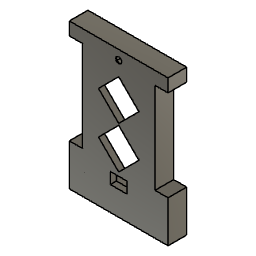
CAO Sablier face avant  v3 -42mm v1 (Autodesk Fusion 360 design; units mm, degrees)
Autodesk Fusion 360 part; units mm, degrees
sketch "Esquisse1" plane through (0, 0, 0) normal (0, 1, 0) x (1, 0, 0)
  line L0 (0, 0) -> (114, 0)
  line L1 (114, 0) -> (114, -150)
  line L2 (114, -150) -> (0, -150)
  line L3 (0, -150) -> (0, 0)
  line L4 (66.6, -23) -> (47.4, -23)
  line L5 (47.4, -23) -> (47.4, -10)
  line L6 (47.4, -10) -> (66.6, -10)
  line L7 (66.6, -10) -> (66.6, -23)
  line L8 (57, -122.669) -> (80.3345, -99.3345)
  line L9 (80.3345, -99.3345) -> (57, -76)
  line L10 (57, -76) -> (33.6655, -99.3345)
  line L11 (33.6655, -99.3345) -> (57, -122.669)
  line L12 (114, -75) -> (0, -75)
  line L13 (33.6655, -50.6655) -> (57, -27.331)
  line L14 (57, -27.331) -> (80.3345, -50.6655)
  line L15 (80.3345, -50.6655) -> (57, -74)
  line L16 (57, -74) -> (33.6655, -50.6655)
  line L17 (114, -135) -> (99, -135)
  line L18 (99, -135) -> (99, -30)
  line L19 (99, -30) -> (114, -30)
  line L20 (114, -30) -> (114, -135)
  line L21 (57, -150) -> (57, 0)
  line L22 (0, -135) -> (15, -135)
  line L23 (15, -135) -> (15, -30)
  line L24 (15, -30) -> (0, -30)
  point P0 (57, -23)
  point P1 (57, -150)
  point P2 (57, -75)
  dimension "d1" = 114
  dimension "d2" = 150
  dimension "d44" = 13
  dimension "d45" = 19.2
  dimension "d46" = 10
  dimension "d48" = 1
  dimension "d49" = 33
  dimension "d159" = 15
  dimension "d160" = 15
  dimension "d161" = 30
  constraint horizontal L0
  constraint vertical L1
  constraint horizontal L2
  constraint vertical L3
  constraint coincident L0.start L3.end
  constraint horizontal L4
  constraint vertical L5
  constraint horizontal L6
  constraint vertical L7
  constraint midpoint L4 P0
  constraint midpoint L2 P1
  constraint vertical P0 P1
  constraint perpendicular L8 L9
  constraint parallel L8 L10
  constraint parallel L9 L11
  constraint vertical L8.start L9.end
  constraint horizontal L8.end L10.end
  constraint vertical P1 L8.start
  constraint coincident L1 L12.start
  constraint coincident L3 L12.end
  constraint perpendicular L3 L12
  constraint midpoint L1 L12.start
  constraint midpoint L12 P2
  constraint symmetric L8.start L12 L13.end
  constraint symmetric L8.end L12 L14.end
  constraint symmetric L9.end L12 L15.end
  constraint symmetric L10.end L12 L13.start
  constraint horizontal L17
  constraint vertical L18
  constraint horizontal L19
  constraint vertical L20
  constraint coincident L1 L17.start
  constraint coincident P1 L21.start
  constraint midpoint L0 L21.end
  constraint symmetric L17.start L21 L22.start
  constraint symmetric L17.end L21 L22.end
  constraint symmetric L18.end L21 L23.end
  constraint symmetric L19.end L21 L24.end
  measures "d1" distance of L1.end L2.end
  measures "d2" distance of L0.end L1.end
  measures "d44" distance of L4.end L5.end
  measures "d45" distance of L4.start L4.end
  measures "d46" distance of L0 L6
  measures "d48" distance of L9.end P2
  measures "d49" distance of L8.start L10.end
  measures "d159" distance of L2 L17
  measures "d160" distance of L18 L20
  measures "d161" distance of L0 L19
extrude "Extrusion14" add sketch "Esquisse1" along normal blind 50 contours L0 L3 L4 L5 L6 L12 L13 L16 L21 L23 L24 | L0 L1 L4 L6 L7 L12 L14 L15 L18 L19 L21 | L3 L12 L23 L24 | L3 L12 L22 L23 | L1 L12 L18 L19 L20 | L2 L3 L10 L11 L12 L21 L22 L23 | L1 L12 L17 L18 L20 | L1 L2 L8 L9 L12 L17 L18 L21 makes body 1
extrude "Extrusion48" cut sketch "Esquisse1" along normal blind 50 contours L1 L12 L17 L18 L20 bodies 1
extrude "Extrusion49" cut sketch "Esquisse1" along normal blind 50 contours L1 L12 L18 L19 L20 bodies 1
extrude "Extrusion50" cut sketch "Esquisse1" along normal blind 50 contours L3 L12 L22 L23 bodies 1
extrude "Extrusion51" cut sketch "Esquisse1" along normal blind 50 contours L3 L12 L23 L24 bodies 1
sketch "Esquisse9" plane through (0, 50, 0) normal (0, 1, 0) x (-1, 0, 0)
  line L0 (-47.4, 10) -> (-66.6, 10)
  line L1 (-66.6, 10) -> (-66.6, 23)
  line L2 (-66.6, 23) -> (-47.4, 23)
  line L3 (-47.4, 23) -> (-47.4, 10)
  line L4 (-80.3345, 50.6655) -> (-57, 74)
  line L5 (-57, 74) -> (-33.6655, 50.6655)
  line L6 (-33.6655, 50.6655) -> (-57, 27.331)
  line L7 (-57, 27.331) -> (-80.3345, 50.6655)
  line L8 (-57, 122.669) -> (-33.6655, 99.3345)
  line L9 (-33.6655, 99.3345) -> (-57, 76)
  line L10 (-57, 76) -> (-80.3345, 99.3345)
  line L11 (-80.3345, 99.3345) -> (-57, 122.669)
  line L12 (0, 150) -> (-114, 150)
  line L13 (-114, 150) -> (-114, 135)
  line L14 (-114, 0) -> (0, 0)
  line L15 (0, 135) -> (0, 150)
  line L16 (-111, 3) -> (-3, 3)
  line L17 (-3, 147) -> (-111, 147)
  line L18 (0, 30) -> (-15, 30)
  line L19 (-15, 30) -> (-15, 135)
  line L20 (-15, 135) -> (0, 135)
  line L21 (-114, 135) -> (-99, 135)
  line L22 (-99, 135) -> (-99, 30)
  line L23 (-99, 30) -> (-114, 30)
  line L24 (-114, 30) -> (-114, 0)
  line L25 (0, 0) -> (0, 30)
  line L26 (-111, 147) -> (-111, 138)
  line L27 (-111, 138) -> (-96, 138)
  line L28 (-96, 138) -> (-96, 27)
  line L29 (-96, 27) -> (-111, 27)
  line L30 (-111, 27) -> (-111, 3)
  line L31 (-3, 147) -> (-3, 138)
  line L32 (-3, 138) -> (-18, 138)
  line L33 (-3, 3) -> (-3, 27)
  line L34 (-3, 27) -> (-18, 27)
  line L35 (-18, 138) -> (-18, 27)
  dimension "d171" = 3
  dimension "d172" = 3
  dimension "d173" = 3
  dimension "d174" = 3
  dimension "d175" = 3
  dimension "d176" = 3
  dimension "d177" = 3
  dimension "d178" = 3
  dimension "d179" = 3
  dimension "d180" = 3
  constraint perpendicular L17 L26
  constraint perpendicular L26 L27
  constraint perpendicular L17 L28
  constraint perpendicular L24 L29
  constraint perpendicular L16 L30
  constraint perpendicular L17 L31
  constraint perpendicular L15 L32
  constraint perpendicular L16 L33
  constraint perpendicular L34 L35
  measures "d171" distance of L24 L30
  measures "d172" distance of L23 L29
  measures "d173" distance of L22 L28
  measures "d174" distance of L21 L27
  measures "d175" distance of L13 L26
  measures "d176" distance of L15 L31
  measures "d177" distance of L20 L32
  measures "d178" distance of L19 L35
  measures "d179" distance of L18 L34
  measures "d180" distance of L25 L33
extrude "Extrusion15" cut sketch "Esquisse9" against normal up to surface (47 mm away) contours L16 L17 L26 L27 L28 L29 L30 L31 L32 L33 L34 L35 bodies 1
sketch "Esquisse10" plane through (0, 3, 0) normal (0, 1, 0) x (-1, 0, 0)
  line L0 (-57, 27.331) -> (-80.3345, 50.6655)
  line L1 (-80.3345, 50.6655) -> (-57, 74)
  line L2 (-57, 74) -> (-33.6655, 50.6655)
  line L3 (-33.6655, 50.6655) -> (-57, 27.331)
  line L4 (-80.3345, 99.3345) -> (-57, 122.669)
  line L5 (-57, 122.669) -> (-33.6655, 99.3345)
  line L6 (-33.6655, 99.3345) -> (-57, 76)
  line L7 (-57, 76) -> (-80.3345, 99.3345)
  line L8 (-47.4, 23) -> (-47.4, 10)
  line L9 (-47.4, 10) -> (-66.6, 10)
  line L10 (-66.6, 10) -> (-66.6, 23)
  line L11 (-66.6, 23) -> (-47.4, 23)
  line L12 (-111, 3) -> (-3, 3)
  line L13 (-3, 147) -> (-111, 147)
  line L14 (-57, 74) -> (-80.3345, 50.6655)
  line L15 (-33.6655, 99.3345) -> (-32.9584, 98.6274)
  line L16 (-32.9584, 98.6274) -> (-57, 74.5858)
  line L17 (-57, 74.5858) -> (-63.364, 80.9497)
  line L18 (-63.364, 80.9497) -> (-62.6569, 81.6569)
  line L19 (-68.6673, 87.6673) -> (-45.3327, 111.0018)
  line L20 (-57, 122.669) -> (-57.7071, 123.3762)
  line L21 (-57.7071, 123.3762) -> (-81.7487, 99.3345)
  line L22 (-81.7487, 99.3345) -> (-75.3848, 92.9706)
  line L23 (-75.3848, 92.9706) -> (-74.6777, 93.6777)
  line L24 (-57, 74) -> (-57.7071, 74.7071)
  line L25 (-57.7071, 74.7071) -> (-81.7487, 50.6655)
  line L26 (-81.7487, 50.6655) -> (-75.3848, 44.3015)
  line L27 (-75.3848, 44.3015) -> (-74.6777, 45.0086)
  line L28 (-68.6673, 38.9982) -> (-45.3327, 62.3327)
  line L29 (-33.6655, 50.6655) -> (-32.9584, 49.9584)
  line L30 (-32.9584, 49.9584) -> (-57, 25.9167)
  line L31 (-57, 25.9167) -> (-63.364, 32.2807)
  line L32 (-63.364, 32.2807) -> (-62.6569, 32.9878)
  line L33 (-57.7071, 123.3762) -> (-57.3536, 123.7297)
  line L34 (-57.3536, 123.7297) -> (-32.6048, 98.981)
  line L35 (-32.6048, 98.981) -> (-32.9584, 98.6274)
  line L36 (-57.7071, 74.7071) -> (-57.3536, 75.0607)
  line L37 (-57.3536, 75.0607) -> (-32.6048, 50.3119)
  line L38 (-32.6048, 50.3119) -> (-32.9584, 49.9584)
  line L39 (-67.6, 24) -> (-46.4, 24)
  line L40 (-46.4, 24) -> (-46.4, 9)
  line L41 (-46.4, 9) -> (-67.6, 9)
  line L42 (-67.6, 9) -> (-67.6, 24)
  line L43 (-45.3327, 62.3327) -> (-44.9792, 62.6863)
  line L44 (-68.6, 3) -> (-97.6, 3)
  line L45 (-97.6, 3) -> (-97.6, 22)
  line L46 (-97.6, 22) -> (-68.6, 22)
  line L47 (-68.6, 22) -> (-68.6, 3)
  line L48 (-96.6, 3) -> (-69.6, 3)
  line L49 (-69.6, 3) -> (-69.6, 21)
  line L50 (-69.6, 21) -> (-96.6, 21)
  line L51 (-96.6, 21) -> (-96.6, 3)
  line L52 (-57, 122.669) -> (-57, 147)
  line L53 (-57, 133) -> (-64, 133)
  line L54 (-64, 133) -> (-64, 145.5)
  line L55 (-64, 145.5) -> (-57, 145.5)
  line L56 (-50, 145.5) -> (-57, 145.5)
  line L57 (-57, 133) -> (-50, 133)
  line L58 (-50, 133) -> (-50, 145.5)
  line L59 (-111, 147) -> (-111, 138)
  line L60 (-111, 138) -> (-96, 138)
  line L61 (-96, 138) -> (-96, 27)
  line L62 (-96, 27) -> (-111, 27)
  line L63 (-111, 27) -> (-111, 3)
  line L64 (-3, 3) -> (-3, 27)
  line L65 (-3, 27) -> (-18, 27)
  line L66 (-18, 27) -> (-18, 138)
  line L67 (-18, 138) -> (-3, 138)
  line L68 (-3, 138) -> (-3, 147)
  line L69 (-32.6048, 98.981) -> (-18, 113.5858)
  circle A0 centre (-5.75, 5.75) radius 1.75
  circle A1 centre (-15.75, 5.75) radius 1.75
  line L70 (-75.3848, 92.9706) -> (-63.364, 80.9497)
  line L71 (-75.3848, 44.3015) -> (-63.364, 32.2807)
  line L72 (-65, 146.5) -> (-49, 146.5)
  line L73 (-49, 146.5) -> (-49, 132)
  line L74 (-49, 132) -> (-65, 132)
  line L75 (-65, 132) -> (-65, 146.5)
  line L76 (-64, 139.25) -> (-50, 139.25)
  circle A2 centre (-57, 139.25) radius 3.5
  dimension "d60" = 1
  dimension "d61" = 9
  dimension "d75" = 9
  dimension "d77" = 1
  dimension "d82" = 0.5
  dimension "d87" = 1
  dimension "d88" = 1
  dimension "d89" = 1
  dimension "d90" = 1
  dimension "d102" = 0.5
  dimension "d113" = 1
  dimension "d114" = 19
  dimension "d115" = 29
  dimension "d116" = 1
  dimension "d117" = 1
  dimension "d118" = 27
  dimension "d119" = 18
  dimension "d127" = 12.5
  dimension "d128" = 7
  dimension "d132" = 1.5
  dimension "d221" = 3.5
  dimension "d222" = 2.75
  dimension "d223" = 2.75
  dimension "d224" = 3.5
  dimension "d225" = 2.75
  dimension "d226" = 10
  dimension "d250" = 1
  dimension "d251" = 1
  dimension "d252" = 1
  dimension "d253" = 1
  dimension "d254" = 7
  constraint coincident L5.end L6.start
  constraint perpendicular L6 L15
  constraint perpendicular L2 L16
  constraint perpendicular L14 L17
  constraint coincident L7 L18.end
  constraint perpendicular L7 L18
  constraint equal L15 L18
  constraint midpoint L7 L19.start
  constraint midpoint L5 L19.end
  constraint symmetric L5.end L19 L4.end
  constraint symmetric L15.end L19 L20.end
  constraint symmetric L16.end L19 L21.end
  constraint symmetric L17.end L19 L22.end
  constraint symmetric L18.end L19 L23.end
  constraint coincident L1.end L2.start
  constraint perpendicular L14 L24
  constraint perpendicular L2 L25
  constraint perpendicular L25 L26
  constraint coincident L0 L27.end
  constraint perpendicular L0 L27
  constraint equal L24 L27
  constraint midpoint L0 L28.start
  constraint midpoint L2 L28.end
  constraint coincident L2.end L3.start
  constraint perpendicular L3 L29
  constraint perpendicular L0 L30
  constraint perpendicular L30 L31
  constraint coincident L0 L32.end
  constraint perpendicular L0 L32
  constraint equal L24 L29
  constraint equal L29 L32
  constraint equal L26 L31
  constraint perpendicular L20 L33
  constraint parallel L5 L34
  constraint parallel L33 L35
  constraint perpendicular L17 L36
  constraint perpendicular L16 L37
  constraint parallel L36 L38
  constraint horizontal L39
  constraint vertical L40
  constraint horizontal L41
  constraint vertical L42
  constraint midpoint L37 L43.end
  constraint horizontal L44
  constraint vertical L45
  constraint horizontal L46
  constraint vertical L47
  constraint coincident L12 L44.start
  constraint horizontal L48
  constraint vertical L49
  constraint horizontal L50
  constraint vertical L51
  constraint midpoint L13 L52.end
  constraint horizontal L53
  constraint vertical L54
  constraint horizontal L55
  constraint coincident L52 L53.start
  constraint symmetric L52 L53.start L57.start
  constraint symmetric L52 L53.end L57.end
  constraint symmetric L52 L54.end L56.start
  constraint symmetric L52 L55.end L56.end
  constraint coincident L66 L69.end
  constraint perpendicular L34 L69
  constraint horizontal L72
  constraint vertical L73
  constraint horizontal L74
  constraint vertical L75
  constraint midpoint L54 L76.start
  constraint midpoint L58 L76.end
  constraint midpoint L76 A2.centre
  measures "d60" distance of L5.end L15.end
  measures "d61" distance of L16.end L17.end
  measures "d75" distance of L25.end L26.end
  measures "d77" distance of L1.end L24.end
  measures "d82" distance of L20.end L33.end
  measures "d87" distance of L11 L39
  measures "d88" distance of L9 L41
  measures "d89" distance of L10 L42
  measures "d90" distance of L8 L40
  measures "d102" distance of L24.end L36.end
  measures "d113" distance of L42 L47
  measures "d114" distance of L44.start L46.end
  measures "d115" distance of L45.end L46.end
  measures "d116" distance of L45 L51
  measures "d117" distance of L46 L50
  measures "d118" distance of L49.end L50.end
  measures "d119" distance of L48.end L49.end
  measures "d127" distance of L53.end L54.end
  measures "d128" distance of L53.start L53.end
  measures "d132" distance of L13 L55
  measures "d221" diameter of A0
  measures "d222" distance of L64 A0.centre
  measures "d223" distance of L12 A0.centre
  measures "d224" diameter of A1
  measures "d225" distance of L12 A1.centre
  measures "d226" distance of A0.centre A1.centre
  measures "d250" distance of L57 L74
  measures "d251" distance of L58 L73
  measures "d252" distance of L55 L72
  measures "d253" distance of L54 L75
  measures "d254" diameter of A2
extrude "Extrusion63" add sketch "Esquisse10" along normal blind 3 contours L0 L27 L32 L71 bodies 1
extrude "Extrusion16" add sketch "Esquisse10" along normal blind 6 contours L0 L1 L2 L14 L28 bodies 1
extrude "Extrusion62" add sketch "Esquisse10" along normal blind 3 separate body contours L7 L18 L23 L70 makes body 2
extrude "Extrusion17" add sketch "Esquisse10" along normal blind 1 contours L6 L7 L15 L16 L17 L18 L36 L37 | L16 L17 L36 L37 bodies 1
extrude "Extrusion18" add 1 faces at (48.9861, 4, 83.0711) along direction (0, 1, 0) blind 6 on bodies 1 bodies 1
extrude "Extrusion19" cut 1 faces at (48.9861, 10, 83.0711) along direction (0, -1, 0) blind 1 on bodies 1 bodies 1
extrude "Extrusion20" add sketch "Esquisse10" along normal blind 6 contours L4 L7 L20 L21 L22 L23 bodies 1
form "Forme1" [no effect]
extrude "Extrusion21" add 1 faces at (68.6673, 9, 54.5546) along direction (0, -1, 0) blind 6 on bodies 1 bodies 1
extrude "Extrusion22" cut 1 faces at (68.6673, 9, 54.5546) along direction (0, -1, 0) blind 12 on bodies 1 bodies 1
extrude "Extrusion23" add sketch "Esquisse10" along normal blind 6 contours L0 L1 L14 L24 L25 L26 L27 bodies 1
extrude "Extrusion24" add sketch "Esquisse10" along normal blind 6 contours L0 L3 L29 L30 L31 L32 bodies 1
extrude "Extrusion25" add sketch "Esquisse10" along normal blind 6 contours L5 L15 L34 L35 L52 | L20 L33 L34 L52 bodies 1
extrude "Extrusion26" add sketch "Esquisse10" along normal blind 6 contours L2 L29 L37 L38 L43 | L2 L16 L17 L24 L36 L37 L43 bodies 1
extrude "Extrusion27" add sketch "Esquisse10" along normal blind 6 contours L39 L40 L41 L42 bodies 1
sketch "Esquisse11" plane through (0, 0, 0) normal (0, 1, 0) x (1, 0, 0)
  line L0 (114, 0) -> (0, 0)
  line L1 (0, 0) -> (0, 18)
  line L2 (0, 18) -> (114, 18)
  line L3 (114, 18) -> (114, 0)
  point P0 (114, 0)
  dimension "d95" = 18
  constraint horizontal L0
  constraint vertical L1
  constraint horizontal L2
  constraint vertical L3
  constraint coincident P0 L0.start
  constraint coincident L0.end L1.start
  measures "d95" distance of L0.end L1.end
extrude "Extrusion28" add sketch "Esquisse11" along normal up to surface (50 mm away) bodies 1
sketch "Esquisse12" plane through (0, 50, 0) normal (0, 1, 0) x (-1, 0, 0)
  line L0 (-3, 3) -> (-111, 3)
  line L1 (-114, 150) -> (-114, 135)
  line L2 (-114, -18) -> (0, -18)
  line L3 (0, 135) -> (0, 150)
  line L4 (-111, 0) -> (-3, 0)
  line L5 (-3, 0) -> (-3, -15)
  line L6 (-3, -15) -> (-111, -15)
  line L7 (-111, -15) -> (-111, 0)
  line L8 (-99, 30) -> (-114, 30)
  line L9 (0, 30) -> (-15, 30)
  line L10 (-3, 27) -> (-3, 3)
  line L11 (-111, 3) -> (-111, 27)
  line L12 (-111, 27) -> (-96, 27)
  line L13 (-96, 27) -> (-96, 138)
  line L14 (-96, 138) -> (-111, 138)
  line L15 (-111, 138) -> (-111, 147)
  line L16 (-111, 147) -> (-3, 147)
  line L17 (-3, 147) -> (-3, 138)
  line L18 (-3, 138) -> (-18, 138)
  line L19 (-18, 138) -> (-18, 27)
  line L20 (-18, 27) -> (-3, 27)
  line L21 (-15, 30) -> (-15, 135)
  line L22 (-15, 135) -> (0, 135)
  line L23 (0, 150) -> (-114, 150)
  line L24 (-114, 135) -> (-99, 135)
  line L25 (-99, 135) -> (-99, 30)
  line L26 (-114, 30) -> (-114, -18)
  line L27 (0, -18) -> (0, 30)
  dimension "d98" = 3
  dimension "d99" = 3
  dimension "d203" = 3
  dimension "d204" = 3
  constraint horizontal L4
  constraint vertical L5
  constraint horizontal L6
  constraint vertical L7
  measures "d98" distance of L0 L4
  measures "d99" distance of L2 L6
  measures "d203" distance of L7 L26
  measures "d204" distance of L5 L27
extrude "Extrusion29" cut sketch "Esquisse12" against normal up to surface (47 mm away) contours L4 L5 L6 L7 bodies 1
extrude "Extrusion30" add 1 faces at (113, 50, 5) along direction (0, 1, 0) blind 10 on bodies 1 bodies 1
extrude "Extrusion31" cut 1 faces at (113, 60, 5) along direction (0, -1, 0) blind 5 on bodies 1 bodies 1
extrude "Extrusion33" add sketch "Esquisse10" along normal blind 47 contours L12 L44 L45 L46 L47 L49 L50 L51 bodies 1
sketch "Esquisse13" plane through (0, 0, 3) normal (0, 0, 1) x (-1, 0, 0)
  line L0 (-96.6, -3) -> (-96.6, -50)
  line L1 (-96.6, -50) -> (-97.6, -50)
  line L2 (-97.6, -50) -> (-97.6, -3)
  line L3 (-97.6, -3) -> (-111, -3)
  line L4 (-111, -55) -> (-3, -55)
  line L5 (-3, -3) -> (-68.6, -3)
  line L6 (-68.6, -3) -> (-68.6, -50)
  line L7 (-68.6, -50) -> (-69.6, -50)
  line L8 (-69.6, -50) -> (-69.6, -3)
  line L9 (-69.6, -3) -> (-96.6, -3)
  line L10 (-109, -55) -> (-99, -55)
  line L11 (-99, -55) -> (-99, -30)
  line L12 (-99, -30) -> (-109, -30)
  line L13 (-109, -30) -> (-109, -55)
  line L14 (-111, -3) -> (-111, -55)
  line L15 (-3, -55) -> (-3, -3)
  dimension "d122" = 10
  dimension "d123" = 25
  constraint horizontal L10
  constraint vertical L11
  constraint horizontal L12
  constraint vertical L13
  constraint coincident L4 L10.start
  measures "d122" distance of L11.end L12.end
  measures "d123" distance of L10.end L11.end
extrude "Extrusion34" cut sketch "Esquisse13" against normal blind 3 contours L4 L10 L11 L12 L13 bodies 1
extrude "Extrusion39" cut 1 faces at (109, 38.3333, 2) along direction (1, 0, 0) blind 2 on bodies 1 bodies 1
extrude "Extrusion40" cut 1 faces at (35.9861, 3, 120.2369) along direction (0, -1, 0) blind 1 on bodies 1 bodies 1
move_body "Déplacer6" bodies 2 to x (1, 0, 0) y (0, 1, 0) z (0, 0, 1) at (0, -1, 0)
extrude "Extrusion41" cut 1 faces at (35.9861, 2, 120.2369) along direction (0, -1, 0) blind 1 on bodies 1 bodies 1
move_body "Déplacer7" bodies 2 to x (1, 0, 0) y (0, 1, 0) z (0, 0, 1) at (0, -1, 0)
extrude "Extrusion42" cut 1 faces at (75, 3, -5) along direction (0, -1, 0) blind 2 on bodies 1 bodies 1
extrude "Extrusion43" cut 1 faces at (87.6, 3, 15) along direction (0, -1, 0) blind 2 on bodies 1 bodies 1
extrude "Extrusion44" cut 1 faces at (48.8683, 9, 34.5199) along direction (0, -1, 0) blind 2 on bodies 1 bodies 1
extrude "Extrusion45" cut 1 faces at (1, 55, 5) along direction (0, -1, 0) blind 2 on bodies 1 bodies 1
extrude "Extrusion46" cut 1 faces at (53.8, 9, 9.3333) along direction (0, -1, 0) blind 2 on bodies 1 bodies 1
extrude "Extrusion47" cut 1 faces at (78.6, 50, 21.6667) along direction (0, -1, 0) blind 2 on bodies 1 bodies 1
extrude "Extrusion68" cut sketch "Esquisse10" against normal blind 5 contours L52 L76 A2 picked at (-55.6052, 141.1132) bodies 1
extrude "Extrusion69" cut sketch "Esquisse10" against normal blind 5 contours L52 L76 A2 | L52 L76 A2 | L52 L76 A2 picked at (-59.3215, 139.084) picked at (-55.6052, 137.3868) picked at (-58.8632, 140.6448) bodies 1
extrude "Extrusion70" add sketch "Esquisse10" along normal blind 8 separate body contours L52 L53 L54 L55 L72 L74 L75 | L52 L56 L57 L58 L72 L73 L74 makes body 3
extrude "Extrusion57" cut 1 faces at (1, 53, 5) along direction (0, -1, 0) blind 10 on bodies 1 bodies 1
extrude "Extrusion58" cut 1 faces at (78.6, 48, 21.6667) along direction (0, -1, 0) blind 10 on bodies 1 bodies 1
extrude "Extrusion59" add 1 faces at (78.6, 38, 21.6667) along direction (0, 1, 0) blind 5 on bodies 1 bodies 1
ref_plane "Plan de construction4" through (5.75, 8, 5.75) normal (0, 1, 0) x (-1, 0, 0)
sketch "Esquisse19" plane through (5.75, 8, 5.75) normal (0, 1, 0) x (1, 0, 0)
  circle A0 centre (10, 0) radius 0.75
  circle A1 centre (0, 0) radius 0.75
  dimension "d235" = 1.5
  dimension "d236" = 1.5
  constraint coincident A1.centre origin
  measures "d235" diameter of A0
  measures "d236" diameter of A1
loft "Lissage3" add profiles "Esquisse19", "Esquisse10" section 1 contours A0 section 2 contours A1 separate body makes body 4
loft "Lissage4" add profiles "Esquisse10", "Esquisse19" section 1 contours A0 section 2 contours A1 separate body makes body 5
move_body "Déplacer4" bodies 4 to x (1, 0, 0) y (0, 1, 0) z (0, 0, 1) at (0, -2, 0)
extrude "Extrusion64" cut 1 faces at (66.8995, 6, 36.759) along direction (0, -1, 0) blind 2 on bodies 1 bodies 1
extrude "Extrusion65" cut 1 faces at (56.8667, 43, 1) along direction (0, -1, 0) blind 21.5 on bodies 1 bodies 1
extrude "Extrusion66" cut 1 faces at (103, 30, 2) along direction (0, -1, 0) blind 8 on bodies 1 bodies 1
extrude "Extrusion67" cut 1 faces at (103, 22, 2) along direction (0, -1, 0) up to surface (0.5 mm away) on bodies 1 bodies 1
move_body "Déplacer8" bodies 5 to x (1, 0, 0) y (0, 1, 0) z (0, 0, 1) at (0, -2, 0)
move_body "Déplacer9" bodies 3 to x (1, 0, 0) y (0, 1, 0) z (0, 0, 1) at (0, -2, 0)
ref_plane "Plan de construction5" through (5.75, 8, 5.75) normal (0, 1, 0) x (-1, 0, 0)
equation "d45 = ( 9.6 * 2 ) * 1 mm"
equation "d95 = 15 mm + 3 mm"
